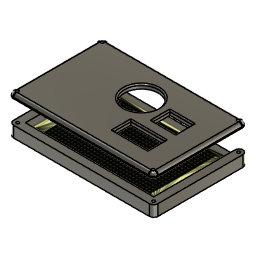
FloppySquare Assembled (Autodesk Fusion 360 design; units mm, degrees)
part number: 2025-07-31-20-16-43-041
part number: 2025-07-31-20-17-13-710
part number: 2025-07-31-20-17-31-222
Autodesk Fusion 360 part; units mm, degrees
sketch "Sketch1" plane through (0, 0, 0) normal (0, 0, 1) x (1, 0, 0) in component "FloppySquare Base (1)"
  line L0 (0, 0) -> (151, 0)
  line L1 (151, 0) -> (151, 100.5)
  line L2 (151, 100.5) -> (0, 100.5)
  line L3 (0, 100.5) -> (0, 0)
  line L4 (-9.5, 0) -> (160.5, 0)
  line L5 (160.5, 0) -> (160.5, 110)
  line L6 (160.5, 110) -> (-9.5, 110)
  line L7 (-9.5, 110) -> (-9.5, 0)
  circle A0 centre (-4.5, 105) radius 1.7
  circle A1 centre (-4.5, 5) radius 1.7
  circle A2 centre (155.5, 5) radius 1.7
  circle A3 centre (155.5, 105) radius 1.7
  circle A4 centre (-4.5, 105) radius 3
  circle A5 centre (-4.5, 5) radius 3
  circle A6 centre (155.5, 5) radius 3
  circle A7 centre (155.5, 105) radius 3
  circle A8 centre (147.5, 13) radius 1.25
  circle A9 centre (147.5, 97) radius 1.25
  circle A10 centre (3.5, 97) radius 1.25
  circle A11 centre (3.5, 13.5) radius 1.25
  dimension "d1_1" = 151
  dimension "d2_1" = 100.5
  dimension "d3_1" = 110
  dimension "d4_1" = 9.5
  dimension "d5_1" = 9.5
  dimension "d6_1" = 3.4
  dimension "d7_1" = 3.4
  dimension "d8_1" = 3.4
  dimension "d9_1" = 3.4
  dimension "d10_1" = 5
  dimension "d11_1" = 5
  dimension "d12_1" = 5
  dimension "d13_1" = 5
  dimension "d14_1" = 5
  dimension "d15_1" = 5
  dimension "d16_1" = 5
  dimension "d17_1" = 5
  dimension "d18_1" = 6
  dimension "d19_1" = 6
  dimension "d20_1" = 6
  dimension "d21_1" = 6
  dimension "d31_1" = 2.5
  dimension "d32_1" = 13
  dimension "d33_1" = 3.5
  dimension "d34_1" = 2.5
  dimension "d35_1" = 3.5
  dimension "d36_1" = 3.5
  dimension "d37_1" = 2.5
  dimension "d38_1" = 3.5
  dimension "d39_1" = 3.5
  dimension "d40_1" = 2.5
  dimension "d41_1" = 13.5
  dimension "d42_1" = 3.5
  constraint horizontal L0
  constraint vertical L1
  constraint horizontal L2
  constraint vertical L3
  constraint coincident L0.start L3.end
  constraint horizontal L4
  constraint vertical L5
  constraint horizontal L6
  constraint vertical L7
  constraint concentric A0 A4
  constraint concentric A1 A5
  constraint concentric A2 A6
  constraint concentric A3 A7
  measures "d1_1" distance of L0.start L0.end
  measures "d2_1" distance of L0.start L2.end
  measures "d3_1" distance of L4.start L6.end
  measures "d4_1" distance of L2 L6
  measures "d5_1" distance of L3 L7
  measures "d6_1" diameter of A0
  measures "d7_1" diameter of A1
  measures "d8_1" diameter of A2
  measures "d9_1" diameter of A3
  measures "d10_1" distance of L6 A0.centre
  measures "d11_1" distance of L7 A0.centre
  measures "d12_1" distance of L4 A1.centre
  measures "d13_1" distance of L7 A1.centre
  measures "d14_1" distance of L4 A2.centre
  measures "d15_1" distance of L5 A2.centre
  measures "d16_1" distance of L6 A3.centre
  measures "d17_1" distance of L5 A3.centre
  measures "d18_1" diameter of A4
  measures "d19_1" diameter of A5
  measures "d20_1" diameter of A6
  measures "d21_1" diameter of A7
  measures "d31_1" diameter of A8
  measures "d32_1" distance of L0 A8.centre
  measures "d33_1" distance of L1 A8.centre
  measures "d34_1" diameter of A9
  measures "d35_1" distance of L2 A9.centre
  measures "d36_1" distance of L1 A9.centre
  measures "d37_1" diameter of A10
  measures "d38_1" distance of L2 A10.centre
  measures "d39_1" distance of L3 A10.centre
  measures "d40_1" diameter of A11
  measures "d41_1" distance of L0 A11.centre
  measures "d42_1" distance of L3 A11.centre
extrude "Extrude1" add sketch "Sketch1" along normal blind 9.9 from surface at 3.1 contours A4 | A5 | A6 | A7 makes body 1 at (157.7981, 6.9284, 9.7) makes body 2 at (152.7356, 103.8347, 9.7) makes body 3 at (-1.5037, 4.8505, 9.7) makes body 4 at (-7.2644, 103.8347, 9.7) in component "FloppySquare Base (1)"
extrude "Extrude2" add sketch "Sketch1" along normal blind 13 contours L1 L2 L3 L4 L5 L6 L7 bodies 1 2 3 4 in component "FloppySquare Base (1)"
extrude "Extrude3" add sketch "Sketch1" along normal blind 3 contours L0 L1 L2 L3 L4 | A8 | A9 | A10 | A11 bodies 1 in component "FloppySquare Base (1)"
fillet "Fillet1" radius 5 4 edges at (160.5, 110, 6.5) (160.5, 0, 6.5) (-9.5, 0, 6.5) (-9.5, 110, 6.5) on bodies 1 in component "FloppySquare Base (1)"
extrude "Extrude4" add sketch "Sketch1" along normal blind 6 contours A8 | A9 | A10 | A11 bodies 1 in component "FloppySquare Base (1)"
fillet "Fillet2" radius 1 4 edges at (146.3346, 96.548, 6) (146.3346, 12.548, 6) (2.3346, 13.048, 6) (2.3346, 96.548, 6) on bodies 1 in component "FloppySquare Base (1)"
fillet "Fillet3" radius 5 2 edges at (0, 0, 8) (151, 0, 8) on bodies 1 in component "FloppySquare Base (1)"
move_body "Move1" bodies 1 to x (-1, 0, 0) y (0, -1, 0) z (0, 0, 1) at (-19, 0, 0) in component "FloppySquare Base (1)"
sketch "Sketch1 (2)" plane through (0, 0, 0) normal (0, 0, 1) x (1, 0, 0) in component "FloppySquare Top (1)"
  line L0 (0, 0) -> (170, 0)
  line L1 (170, 0) -> (170, 110)
  line L2 (170, 110) -> (0, 110)
  line L3 (0, 110) -> (0, 0)
  circle A0 centre (5, 105) radius 1.7
  circle A1 centre (5, 5) radius 1.7
  circle A2 centre (165, 105) radius 1.7
  circle A3 centre (165, 5) radius 1.7
  line L4 (141.5, 75) -> (114.5, 75)
  line L5 (114.5, 75) -> (114.5, 55)
  line L6 (114.5, 55) -> (141.5, 55)
  line L7 (141.5, 55) -> (141.5, 75)
  circle A4 centre (85, 71) radius 20
  line L8 (141.5, 22) -> (101.5, 22)
  line L9 (101.5, 22) -> (101.5, 42)
  line L10 (101.5, 42) -> (141.5, 42)
  line L11 (141.5, 42) -> (141.5, 22)
  dimension "d1_2" = 170
  dimension "d2_2" = 110
  dimension "d3_2" = 3.4
  dimension "d4_2" = 3.4
  dimension "d5_2" = 3.4
  dimension "d6_2" = 3.4
  dimension "d7_2" = 5
  dimension "d8_2" = 5
  dimension "d9_2" = 5
  dimension "d10_2" = 5
  dimension "d11_2" = 5
  dimension "d12_2" = 5
  dimension "d13_2" = 5
  dimension "d14_2" = 5
  dimension "d15_2" = 27
  dimension "d16_2" = 20
  dimension "d17_2" = 28.5
  dimension "d18_2" = 35
  dimension "d19_2" = 40
  dimension "d20_2" = 85
  dimension "d21_2" = 39
  dimension "d22_2" = 40
  dimension "d23_2" = 20
  dimension "d24_2" = 22
  dimension "d25_2" = 28.5
  constraint horizontal L0
  constraint vertical L1
  constraint horizontal L2
  constraint vertical L3
  constraint coincident L0.start L3.end
  constraint horizontal L4
  constraint vertical L5
  constraint horizontal L6
  constraint vertical L7
  constraint horizontal L8
  constraint vertical L9
  constraint horizontal L10
  constraint vertical L11
  measures "d1_2" distance of L0.start L0.end
  measures "d2_2" distance of L0.start L2.end
  measures "d3_2" diameter of A0
  measures "d4_2" diameter of A1
  measures "d5_2" diameter of A2
  measures "d6_2" diameter of A3
  measures "d7_2" distance of L0 A3.centre
  measures "d8_2" distance of L1 A3.centre
  measures "d9_2" distance of L2 A2.centre
  measures "d10_2" distance of L1 A2.centre
  measures "d11_2" distance of L2 A0.centre
  measures "d12_2" distance of L3 A0.centre
  measures "d13_2" distance of L0 A1.centre
  measures "d14_2" distance of L3 A1.centre
  measures "d15_2" distance of L4.start L4.end
  measures "d16_2" distance of L4.start L6.end
  measures "d17_2" distance of L1 L7
  measures "d18_2" distance of L2 L4
  measures "d19_2" diameter of A4
  measures "d20_2" distance of L3 A4.centre
  measures "d21_2" distance of L2 A4.centre
  measures "d22_2" distance of L8.start L8.end
  measures "d23_2" distance of L8.start L10.end
  measures "d24_2" distance of L0 L8
  measures "d25_2" distance of L1 L11
extrude "Extrude1'" add sketch "Sketch1 (2)" along normal blind 5 separate body makes body 5 in component "FloppySquare Top (1)"
fillet "Fillet1'" radius 5 4 edges at (0, 110, 2.5) (0, 0, 2.5) (170, 0, 2.5) (170, 110, 2.5) on bodies 5 in component "FloppySquare Top (1)"
fillet "Fillet2'" radius 3.5 8 edges at (1.4645, 108.5355, 5) (0, 55, 5) (1.4645, 1.4645, 5) (85, 0, 5) (168.5355, 1.4645, 5) (170, 55, 5) (168.5355, 108.5355, 5) (85, 110, 5) on bodies 5 in component "FloppySquare Top (1)"
fillet "Fillet3'" radius 1.5 9 edges at (141.5, 65, 5) (128, 55, 5) (114.5, 65, 5) (128, 75, 5) (121.5, 42, 5) (141.5, 32, 5) (101.5, 32, 5) (121.5, 22, 5) (66.3535, 78.2323, 5) on bodies 5 in component "FloppySquare Top (1)"
other "Base Mesh Feature1"
other "Modify1"
component "FloppySquare Base (1)" placed x (1, 0, 0) y (0, 1, 0) z (0, 0, 1) at (0, 0, 0)
component "FloppySquare Top (1)" placed x (1, 0, 0) y (0, 1, 0) z (0, 0, 1) at (0, 0, 0)
